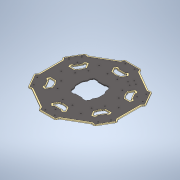
# Autodesk Inventor part: FRAME ATAS
Saved by Autodesk Inventor 2020.2 (Build 242310000, 310)
## iProperties
Created: 2020-03-27
Part Number: FRAME ATAS
Material: Generic
Document SubType Name: Modeling
Designer: Muhyidin
Density: 1 g/cm^3
Appearance: Carbon Fiber
Author: Muhyidin
Autodesk Inventor part; units mm, degrees
(part 1 of 2)
ref_plane "YZ Plane" through (0, 0, 0) normal (1, 0, 0) x (0, 1, 0)
ref_plane "XZ Plane" through (0, 0, 0) normal (0, 1, 0) x (-1, 0, 0)
ref_plane "XY Plane" through (0, 0, 0) normal (0, 0, 1) x (1, 0, 0)
sketch "Sketch1" plane through (0, 0, 0) normal (0, 1, 0) x (-1, 0, 0)
  circle A0 centre (15.3999, -131.0001) radius 1.6
  circle A1 centre (-15.4001, -131) radius 1.6
  line L0 (-50.3385, -87.1889) -> (-60.4808, -89.9065)
  circle A2 centre (-60.4808, -89.9065) radius 1.5
  line L1 (-50.3385, -87.1889) -> (-40.1963, -84.4713)
  line L2 (-50.3385, -87.1889) -> (-47.6209, -97.3311)
  line L3 (-50.3385, -87.1889) -> (-53.0561, -77.0467)
  circle A3 centre (-53.0561, -77.0467) radius 1.5
  circle A4 centre (-40.1963, -84.4713) radius 1.5
  circle A5 centre (-47.6209, -97.3311) radius 1.5
  line L4 (68.5102, -57.3368) -> (53.5102, -83.3176)
  line L5 (83.9102, -30.6632) -> (98.9102, -4.6824)
  line L6 (-68.5102, 57.3368) -> (-53.5102, 83.3176)
  line L7 (-83.9102, 30.6632) -> (-98.9102, 4.6824)
  line L8 (-83.9102, 30.6632) -> (-53.9102, 30.6632) construction
  circle A6 centre (98.9102, -4.6824) radius 1.6
  circle A7 centre (53.5102, -83.3176) radius 1.6
  circle A8 centre (-98.9102, 4.6824) radius 1.6
  circle A9 centre (-53.5102, 83.3176) radius 1.6
  line L9 (53.5102, -83.3176) -> (68.5102, -83.3176) construction
  circle A10 centre (0, 113) radius 1.6
  line L10 (76.2102, -44) -> (97.8609, -56.5)
  line L11 (76.2102, -44) -> (101.2102, -44) construction
  circle A11 centre (97.8609, -56.5) radius 1.6
  line L12 (-76.2102, -44) -> (-97.8609, -56.5)
  line L13 (-76.2102, -44) -> (-51.2102, -44) construction
  circle A12 centre (-97.8609, -56.5) radius 1.6
  line L14 (25, -145) -> (60, -145) construction
  line L15 (0, -138) -> (25, -138)
  line L16 (0, -138) -> (25, -138) construction
  line L17 (0, -138) -> (-25, -138)
  line L18 (0, -138) -> (25, -138) construction
  line L19 (15.4, -138) -> (22.4, -138) construction
  line L20 (-15.4, -138.0001) -> (-8.4, -138.0001) construction
  line L21 (-25, -138) -> (4.9988, -138) construction
  line L22 (-92.0115, -90.6506) -> (-87.0115, -90.6506) construction
  line L23 (-25, -138) -> (-5.0008, -138) construction
  line L24 (-25, -138) -> (-28.4202, -128.6031)
  line L25 (-25, -138) -> (-15, -138) construction
  line L26 (25, -138) -> (28.4201, -128.6031)
  line L27 (132.0114, -47.3494) -> (125.5835, -39.689)
  line L28 (107.0114, -90.6507) -> (97.1633, -88.9142)
  line L29 (111.8115, -82.3369) -> (115.3115, -76.2747) construction
  line L30 (107.0114, -90.6507) -> (117.011, -73.3308) construction
  line L31 (119.5114, -69) -> (107.0114, -90.6507)
  line L32 (107.0114, -90.6507) -> (122.0108, -64.6709) construction
  line L33 (119.5114, -69) -> (132.0114, -47.3494)
  line L34 (119.5114, -69) -> (132.0114, -47.3494) construction
  line L35 (119.5114, -69) -> (132.0114, -47.3494) construction
  circle A13 centre (121.1493, -52.1634) radius 1.6
  circle A14 centre (105.7492, -78.8369) radius 1.6
  line L36 (107.0114, 90.6505) -> (97.1634, 88.914)
  line L37 (132.0114, 47.3493) -> (125.5835, 39.6888)
  line L38 (127.2115, 55.6631) -> (123.7115, 61.7253) construction
  line L39 (132.0114, 47.3493) -> (122.0118, 64.6691) construction
  line L40 (119.5114, 68.9999) -> (132.0114, 47.3493)
  line L41 (132.0114, 47.3493) -> (117.012, 73.329) construction
  line L42 (119.5114, 68.9999) -> (107.0114, 90.6505)
  line L43 (119.5114, 68.9999) -> (107.0114, 90.6505) construction
  line L44 (119.5114, 68.9999) -> (107.0114, 90.6505) construction
  circle A15 centre (105.7494, 78.8366) radius 1.6
  circle A16 centre (121.1493, 52.163) radius 1.6
  line L45 (-25.0001, 137.9998) -> (-28.4202, 128.6029)
  line L46 (24.9999, 137.9998) -> (28.4202, 128.6029)
  line L47 (15.4, 137.9999) -> (8.4, 137.9999) construction
  line L48 (24.9999, 137.9998) -> (5.0007, 137.9998) construction
  line L49 (-0.0001, 137.9998) -> (24.9999, 137.9998)
  line L50 (24.9999, 137.9998) -> (-4.9989, 137.9998) construction
  line L51 (-0.0001, 137.9998) -> (-25.0001, 137.9998)
  line L52 (-0.0001, 137.9998) -> (-25.0001, 137.9998) construction
  line L53 (-0.0001, 137.9998) -> (-25.0001, 137.9998) construction
  circle A17 centre (-15.3999, 130.9999) radius 1.6
  circle A18 centre (15.4, 130.9999) radius 1.6
  line L54 (-132.0115, 47.3492) -> (-125.5836, 39.6889)
  line L55 (-107.0115, 90.6505) -> (-97.1634, 88.914)
  line L56 (-111.8115, 82.3367) -> (-115.3115, 76.2745) construction
  line L57 (-107.0115, 90.6505) -> (-117.0111, 73.3307) construction
  line L58 (-119.5115, 68.9999) -> (-107.0115, 90.6505)
  line L59 (-107.0115, 90.6505) -> (-122.0109, 64.6707) construction
  line L60 (-119.5115, 68.9999) -> (-132.0115, 47.3492)
  line L61 (-119.5115, 68.9999) -> (-132.0115, 47.3492) construction
  line L62 (-119.5115, 68.9999) -> (-132.0115, 47.3492) construction
  circle A19 centre (-121.1493, 52.1632) radius 1.6
  circle A20 centre (-105.7493, 78.8367) radius 1.6
  line L63 (-107.0114, -90.6507) -> (-97.1634, -88.9142)
  line L64 (-132.0114, -47.3494) -> (-125.5836, -39.689)
  line L65 (-127.2115, -55.6633) -> (-123.7115, -61.7255) construction
  line L66 (-132.0114, -47.3494) -> (-122.0118, -64.6693) construction
  line L67 (-119.5114, -69.0001) -> (-132.0114, -47.3494)
  line L68 (-132.0114, -47.3494) -> (-117.012, -73.3292) construction
  line L69 (-119.5114, -69.0001) -> (-107.0114, -90.6507)
  line L70 (-119.5114, -69.0001) -> (-107.0114, -90.6507) construction
  line L71 (-119.5114, -69.0001) -> (-107.0114, -90.6507) construction
  circle A21 centre (-105.7494, -78.8368) radius 1.6
  circle A22 centre (-121.1493, -52.1632) radius 1.6
  line L72 (-28.4202, -128.6031) -> (-97.1634, -88.9142)
  line L73 (97.1633, -88.9142) -> (28.4201, -128.6031)
  line L74 (125.5835, 39.6888) -> (125.5835, -39.689)
  line L75 (28.4202, 128.6029) -> (97.1634, 88.914)
  line L76 (-97.1634, 88.914) -> (-28.4202, 128.6029)
  line L77 (-125.5836, -39.689) -> (-125.5836, 39.6889)
  line L78 (-15.4, -131) -> (42.1, -131) construction
  line L79 (36.5897, -0.0001) -> (36.5897, -10.9001)
  line L80 (36.5897, -0.0001) -> (47.4897, -0.0001) construction
  line L81 (36.5897, -10.9001) -> (30.2097, -21.9505)
  line L82 (36.5897, -10.9001) -> (49.3497, -10.9001) construction
  line L83 (30.2097, -21.9505) -> (30.2097, -30.6505)
  line L84 (30.2097, -21.9505) -> (38.9097, -21.9505) construction
  line L85 (30.2097, -30.6505) -> (23.4386, -38.72)
  line L86 (30.2097, -30.6505) -> (40.7437, -30.6505) construction
  line L87 (23.4386, -38.72) -> (12.9386, -38.72)
  line L88 (12.9386, -38.72) -> (11.0102, -36.4219)
  line L89 (0, -83.2026) -> (6, -83.2026)
  line L90 (6, -83.2026) -> (8.5, -83.2026) construction
  line L91 (6, -83.2026) -> (7.9151, -84.8096)
  line L92 (6, -83.2026) -> (8.5, -83.2026) construction
  line L93 (7.9151, -84.8096) -> (14.9151, -84.8096)
  line L94 (14.9151, -84.8096) -> (24.9151, -102.1301)
  line L95 (14.9151, -90.5569) -> (34.9151, -90.5569) construction
  line L96 (24.9151, -102.1301) -> (19.1301, -109.0245)
  line L97 (24.9151, -115.3493) -> (33.9151, -115.3493) construction
  line L98 (19.1301, -109.0245) -> (13.35, -109.0245)
  line L99 (19.1301, -114.7719) -> (24.9101, -114.7719) construction
  line L100 (13.35, -109.0245) -> (11.1, -105.1274)
  line L101 (13.35, -109.0245) -> (17.85, -109.0245) construction
  line L102 (11.1, -105.1274) -> (0, -105.1274)
  line L103 (0, -83.2026) -> (-6, -83.2026)
  line L104 (-6, -83.2026) -> (-8.5, -83.2026) construction
  line L105 (-6, -83.2026) -> (-7.9151, -84.8096)
  line L106 (-6, -83.2026) -> (-8.5, -83.2026) construction
  line L107 (-7.9151, -84.8096) -> (-14.9151, -84.8096)
  line L108 (-14.9151, -84.8096) -> (-24.9151, -102.1301)
  line L109 (-14.9151, -90.557) -> (-34.9151, -90.557) construction
  line L110 (-24.9151, -102.1301) -> (-19.13, -109.0245)
  line L111 (-19.13, -109.0245) -> (-13.35, -109.0245)
  line L112 (-19.13, -114.7719) -> (-24.91, -114.7719) construction
  line L113 (-13.35, -109.0245) -> (-11.1, -105.1274)
  line L114 (-13.35, -109.0245) -> (-17.85, -109.0245) construction
  line L115 (-11.1, -105.1274) -> (0, -105.1274)
  line L116 (0, -88.9499) -> (0, -36.4219)
  line L117 (0, -86.2026) -> (5.9999, -86.2026)
  line L118 (5.9999, -86.2026) -> (7.532, -87.4882)
  line L119 (5.9999, -86.2026) -> (7.9999, -86.2026) construction
  line L120 (7.532, -87.4882) -> (12.532, -87.4882)
  line L121 (12.532, -87.4882) -> (20.032, -100.4785)
  line L122 (20.032, -100.4785) -> (16.8181, -104.3088)
  line L123 (16.8181, -104.3088) -> (13.8181, -104.3088)
  line L124 (13.8181, -104.3088) -> (12.5681, -102.1437)
  line L125 (12.5681, -102.1437) -> (0, -102.1437)
  line L126 (0, -86.2026) -> (-6, -86.2026)
  line L127 (-6, -86.2026) -> (-7.5321, -87.4882)
  line L128 (-6, -86.2026) -> (-8, -86.2026) construction
  line L129 (-7.5321, -87.4882) -> (-12.5321, -87.4882)
  line L130 (-12.5321, -87.4882) -> (-20.0321, -100.4785)
  line L131 (-20.0321, -100.4785) -> (-16.8181, -104.3088)
  line L132 (-16.8181, -104.3088) -> (-13.8181, -104.3088)
  line L133 (-13.8181, -104.3088) -> (-12.5681, -102.1437)
  line L134 (-12.5681, -102.1437) -> (0, -102.1437)
  line L135 (0, -138) -> (0, -141)
  line L136 (0, -138) -> (3, -138) construction
  line L137 (-25, -138) -> (-22, -138) construction
  line L138 (-25, -138) -> (-20, -138) construction
  line L139 (0, -141) -> (-27.5173, -141)
  line L140 (0, -141) -> (27.5173, -141) construction
  line L141 (-27.5173, -141) -> (-13.8071, -141) construction
  line L142 (-28.4202, -128.6031) -> (-34.2721, -128.6031)
  line L143 (-28.4202, -128.6031) -> (-22.5683, -128.6031) construction
  line L144 (-107.0114, -90.6507) -> (-104.0114, -90.6507) construction
  line L145 (-27.5173, -141) -> (-30.9375, -131.6031)
  line L146 (-27.5173, -141) -> (-17.5173, -141) construction
  line L147 (0, -141) -> (27.5173, -141)
  line L148 (27.5173, -141) -> (13.8071, -141) construction
  line L149 (27.5173, -141) -> (30.9375, -131.6031)
  line L150 (108.3508, -94.3307) -> (98.5028, -92.5942)
  line L151 (122.1095, -70.5) -> (108.3508, -94.3307)
  line L152 (122.1095, -70.5) -> (135.8681, -46.6693) construction
  line L153 (122.1095, -70.5) -> (135.8681, -46.6693)
  line L154 (135.8681, -46.6693) -> (129.4403, -39.0089)
  line L155 (135.8681, 46.6692) -> (129.4402, 39.0088)
  line L156 (122.1095, 70.4999) -> (135.8681, 46.6692)
  line L157 (122.1095, 70.4999) -> (108.3508, 94.3306) construction
  line L158 (122.1095, 70.4999) -> (108.3508, 94.3306)
  line L159 (108.3508, 94.3306) -> (98.5027, 92.5941)
  line L160 (27.5172, 140.9998) -> (30.9374, 131.6029)
  line L161 (-0.0001, 140.9998) -> (27.5172, 140.9998)
  line L162 (-0.0001, 140.9998) -> (-27.5173, 140.9998) construction
  line L163 (-0.0001, 140.9998) -> (-27.5173, 140.9998)
  line L164 (-27.5173, 140.9998) -> (-30.9376, 131.6029)
  line L165 (-108.3509, 94.3305) -> (-98.5028, 92.5941)
  line L166 (-122.1095, 70.4999) -> (-108.3509, 94.3305)
  line L167 (-122.1095, 70.4999) -> (-135.8682, 46.6692) construction
  line L168 (-122.1095, 70.4999) -> (-135.8682, 46.6692)
  line L169 (-135.8682, 46.6692) -> (-129.4403, 39.0087)
  line L170 (-135.8682, -46.6694) -> (-129.4403, -39.0089)
  line L171 (-122.1095, -70.5001) -> (-135.8682, -46.6694)
  line L172 (-122.1095, -70.5001) -> (-108.3509, -94.3307) construction
  line L173 (-122.1095, -70.5001) -> (-108.3509, -94.3307)
  line L174 (-108.3509, -94.3307) -> (-98.5028, -92.5943)
  line L175 (-30.9375, -131.6031) -> (-98.5028, -92.5943)
  line L176 (98.5028, -92.5942) -> (30.9375, -131.6031)
  line L177 (129.4402, 39.0088) -> (129.4403, -39.0089)
  line L178 (30.9374, 131.6029) -> (98.5027, 92.5941)
  line L179 (-98.5028, 92.5941) -> (-30.9376, 131.6029)
  line L180 (-129.4403, -39.0089) -> (-129.4403, 39.0087)
  line L181 (11.0102, -36.4219) -> (0, -36.4219)
  line L182 (-36.5897, -0.0001) -> (-36.5897, -10.9001)
  line L183 (-36.5897, -10.9001) -> (-30.2097, -21.9505)
  line L184 (-36.5897, -10.9001) -> (-49.3497, -10.9001) construction
  line L185 (-30.2097, -21.9505) -> (-30.2097, -30.6505)
  line L186 (-30.2097, -21.9505) -> (-38.9097, -21.9505) construction
  line L187 (-30.2097, -30.6505) -> (-23.4386, -38.72)
  line L188 (-23.4386, -38.72) -> (-12.9386, -38.72)
  line L189 (-12.9386, -38.72) -> (-11.0102, -36.4219)
  line L190 (-11.0102, -36.4219) -> (0, -36.4219)
  line L191 (36.5897, -0.0001) -> (36.5897, 10.8999)
  line L192 (36.5897, 10.8999) -> (30.2097, 21.9504)
  line L193 (36.5897, 10.8999) -> (49.3497, 10.8999) construction
  line L194 (30.2097, 21.9504) -> (30.2097, 30.6504)
  line L195 (30.2097, 21.9504) -> (38.9097, 21.9504) construction
  line L196 (30.2097, 30.6504) -> (23.4386, 38.7199)
  line L197 (23.4386, 38.7199) -> (12.9386, 38.7199)
  line L198 (12.9386, 38.7199) -> (11.0102, 36.4218)
  line L199 (11.0102, 36.4218) -> (0, 36.4218)
  line L200 (-23.4386, 38.7199) -> (-12.9386, 38.7199)
  line L201 (-30.2097, 30.6504) -> (-23.4386, 38.7199)
  line L202 (-11.0102, 36.4218) -> (0, 36.4218)
  line L203 (-12.9386, 38.7199) -> (-11.0102, 36.4218)
  line L204 (-30.2097, 21.9504) -> (-30.2097, 30.6504)
  line L205 (-30.2097, 21.9504) -> (-38.9097, 21.9504) construction
  line L206 (-36.5897, 10.8999) -> (-30.2097, 21.9504)
  line L207 (-36.5897, 10.8999) -> (-49.3497, 10.8999) construction
  line L208 (-36.5897, -0.0001) -> (-36.5897, 10.8999)
  line L209 (-15.4, -131) -> (-15.4, -73.5)
  line L210 (-15.4, -131) -> (42.1, -131) construction
  line L211 (15.3999, -131.0001) -> (15.3999, -73.5001)
  line L212 (15.3999, -73.5001) -> (15.9999, -73.5001)
  line L213 (15.3999, -73.5001) -> (15.9999, -73.5001) construction
  circle A23 centre (15.9999, -73.5001) radius 1.65
  line L214 (-15.4, -73.5) -> (-16.036, -73.5)
  circle A24 centre (-16.0361, -73.5) radius 1.65
  circle A25 centre (55.6348, -50.6377) radius 1.65
  circle A26 centre (71.6528, -22.8937) radius 1.65
  circle A27 centre (71.6708, 22.8623) radius 1.65
  circle A28 centre (55.6529, 50.6063) radius 1.65
  circle A29 centre (16.036, 73.4999) radius 1.65
  circle A30 centre (-15.9999, 73.4999) radius 1.65
  circle A31 centre (-55.6348, 50.6375) radius 1.65
  circle A32 centre (-71.6529, 22.8936) radius 1.65
  circle A33 centre (-71.6709, -22.8624) radius 1.65
  circle A34 centre (-55.6529, -50.6064) radius 1.65
  line L215 (85.4929, -62.1766) -> (91.0429, -52.5637)
  line L216 (82.1749, -61.9562) -> (88.4589, -51.0719)
  line L217 (94.743, -40.1876) -> (88.4589, -51.0719)
  line L218 (96.5929, -42.9508) -> (91.0429, -52.5637)
  line L219 (101.0929, -42.9508) -> (96.5929, -42.9508)
  line L220 (97.243, -40.1876) -> (94.743, -40.1876)
  line L221 (100.9047, -29.488) -> (103.9829, -37.9452)
  line L222 (101.0929, -42.9508) -> (103.3429, -39.0537) construction
  line L223 (103.9829, -37.9452) -> (101.0929, -42.9508)
  line L224 (98.743, -37.5895) -> (97.243, -40.1876)
  line L225 (97.0329, -32.8911) -> (98.743, -37.5895)
  line L226 (80.9047, -29.488) -> (100.9047, -29.488)
  line L227 (82.0329, -32.8911) -> (97.0329, -32.8911)
  line L228 (79.5329, -37.2212) -> (82.0329, -32.8911)
  line L229 (77.4047, -35.5501) -> (80.9047, -29.488)
  line L230 (77.6535, -37.9052) -> (79.5329, -37.2212)
  line L231 (75.0555, -36.4052) -> (77.4047, -35.5501)
  line L232 (75.0555, -36.4052) -> (76.3055, -34.2401) construction
  line L233 (75.0555, -36.4052) -> (76.3055, -34.2401) construction
  line L234 (72.0555, -41.6013) -> (75.0555, -36.4052)
  line L235 (77.6535, -37.9052) -> (78.6535, -36.1732) construction
  line L236 (74.6535, -43.1013) -> (77.6535, -37.9052)
  line L237 (69.0555, -46.7975) -> (67.8055, -48.9625) construction
  line L238 (69.0555, -46.7975) -> (67.8055, -48.9625) construction
  line L239 (72.0555, -41.6013) -> (69.0555, -46.7975)
  line L240 (74.6535, -43.1013) -> (71.6536, -48.2974)
  line L241 (69.0555, -46.7975) -> (69.4896, -49.2595)
  line L242 (71.6536, -48.2974) -> (70.6536, -50.0295) construction
  line L243 (71.6536, -48.2974) -> (72.0008, -50.2671)
  line L244 (69.4896, -49.2595) -> (65.9896, -55.3217)
  line L245 (72.0008, -50.2671) -> (69.5008, -54.5972)
  line L246 (69.5008, -54.5972) -> (77.0008, -67.5876)
  line L247 (65.9896, -55.3217) -> (75.9896, -72.6422)
  line L248 (70.967, -58.1954) -> (60.967, -75.5159) construction
  line L249 (81.9249, -66.7193) -> (83.4249, -64.1213)
  line L250 (84.8529, -71.0793) -> (87.7429, -66.0737)
  line L251 (87.7429, -66.0737) -> (85.4929, -69.9708) construction
  line L252 (87.7429, -66.0737) -> (85.4929, -62.1766)
  line L253 (83.4249, -64.1213) -> (82.1749, -61.9562)
  line L254 (77.0008, -67.5876) -> (81.9249, -66.7193)
  line L255 (75.9896, -72.6422) -> (84.8529, -71.0793)
  line L256 (96.5929, 42.9507) -> (91.0429, 52.5636)
  line L257 (94.743, 40.1874) -> (88.4589, 51.0717)
  line L258 (82.1749, 61.956) -> (88.4589, 51.0717)
  line L259 (85.4929, 62.1765) -> (91.0429, 52.5636)
  line L260 (87.7429, 66.0736) -> (85.4929, 62.1765)
  line L261 (83.4249, 64.1211) -> (82.1749, 61.956)
  line L262 (75.9896, 72.642) -> (84.8529, 71.0793)
  line L263 (87.7429, 66.0736) -> (85.4929, 69.9707) construction
  line L264 (84.8529, 71.0793) -> (87.7429, 66.0736)
  line L265 (81.9249, 66.7192) -> (83.4249, 64.1211)
  line L266 (77.0008, 67.5874) -> (81.9249, 66.7192)
  line L267 (65.9896, 55.3215) -> (75.9896, 72.642)
  line L268 (69.5008, 54.597) -> (77.0008, 67.5874)
  line L269 (72.0008, 50.2669) -> (69.5008, 54.597)
  line L270 (69.4896, 49.2593) -> (65.9896, 55.3215)
  line L271 (71.6536, 48.2973) -> (72.0008, 50.2669)
  line L272 (69.0555, 46.7973) -> (69.4896, 49.2593)
  line L273 (69.0555, 46.7973) -> (67.8054, 48.9624) construction
  line L274 (69.0555, 46.7973) -> (67.8055, 48.9624) construction
  line L275 (72.0555, 41.6012) -> (69.0555, 46.7973)
  line L276 (71.6536, 48.2973) -> (70.6536, 50.0293) construction
  line L277 (74.6535, 43.1012) -> (71.6536, 48.2973)
  line L278 (75.0555, 36.4051) -> (76.3055, 34.24) construction
  line L279 (75.0555, 36.4051) -> (76.3055, 34.24) construction
  line L280 (72.0555, 41.6012) -> (75.0555, 36.4051)
  line L281 (74.6535, 43.1012) -> (77.6535, 37.9051)
  line L282 (75.0555, 36.4051) -> (77.4047, 35.55)
  line L283 (77.6535, 37.9051) -> (78.6535, 36.173) construction
  line L284 (77.6535, 37.9051) -> (79.5329, 37.221)
  line L285 (77.4047, 35.55) -> (80.9047, 29.4879)
  line L286 (79.5329, 37.221) -> (82.0329, 32.8909)
  line L287 (82.0329, 32.8909) -> (97.0329, 32.8909)
  line L288 (80.9047, 29.4879) -> (100.9047, 29.4879)
  line L289 (85.8821, 32.3615) -> (95.8821, 15.041) construction
  line L290 (98.743, 37.5894) -> (97.243, 40.1874)
  line L291 (103.9829, 37.9451) -> (101.0929, 42.9507)
  line L292 (101.0929, 42.9507) -> (103.3429, 39.0536) construction
  line L293 (101.0929, 42.9507) -> (96.5929, 42.9507)
  line L294 (97.243, 40.1874) -> (94.743, 40.1874)
  line L295 (97.0329, 32.8909) -> (98.743, 37.5894)
  line L296 (100.9047, 29.4879) -> (103.9829, 37.9451)
  line L297 (11.0999, 105.1272) -> (-0.0001, 105.1272)
  line L298 (12.5681, 102.1435) -> (0, 102.1435)
  line L299 (-12.5681, 102.1435) -> (0, 102.1435)
  line L300 (-11.1001, 105.1272) -> (-0.0001, 105.1272)
  line L301 (-13.3501, 109.0244) -> (-11.1001, 105.1272)
  line L302 (-13.8181, 104.3086) -> (-12.5681, 102.1435)
  line L303 (-24.9151, 102.1299) -> (-19.1301, 109.0244)
  line L304 (-13.3501, 109.0244) -> (-17.8501, 109.0244) construction
  line L305 (-19.1301, 109.0244) -> (-13.3501, 109.0244)
  line L306 (-16.8181, 104.3086) -> (-13.8181, 104.3086)
  line L307 (-20.0321, 100.4784) -> (-16.8181, 104.3086)
  line L308 (-14.9151, 84.8094) -> (-24.9151, 102.1299)
  line L309 (-12.5321, 87.488) -> (-20.0321, 100.4784)
  line L310 (-7.5321, 87.488) -> (-12.5321, 87.488)
  line L311 (-7.9151, 84.8094) -> (-14.9151, 84.8094)
  line L312 (-6, 86.2024) -> (-7.5321, 87.488)
  line L313 (-6, 83.2024) -> (-7.9151, 84.8094)
  line L314 (-6, 83.2024) -> (-8.5001, 83.2024) construction
  line L315 (-6, 83.2024) -> (-8.5, 83.2024) construction
  line L316 (0, 83.2024) -> (-6, 83.2024)
  line L317 (-6, 86.2024) -> (-8, 86.2024) construction
  line L318 (0, 86.2024) -> (-6, 86.2024)
  line L319 (5.9999, 83.2025) -> (8.4999, 83.2025) construction
  line L320 (5.9999, 83.2025) -> (8.4999, 83.2025) construction
  line L321 (0, 83.2024) -> (5.9999, 83.2025)
  line L322 (0, 86.2024) -> (5.9999, 86.2024)
  line L323 (5.9999, 83.2025) -> (7.915, 84.8094)
  line L324 (5.9999, 86.2024) -> (7.9999, 86.2024) construction
  line L325 (5.9999, 86.2024) -> (7.532, 87.488)
  line L326 (7.915, 84.8094) -> (14.915, 84.8094)
  line L327 (7.532, 87.488) -> (12.532, 87.488)
  line L328 (12.532, 87.488) -> (20.032, 100.4784)
  line L329 (14.915, 84.8094) -> (24.915, 102.13)
  line L330 (14.915, 90.5568) -> (34.915, 90.5568) construction
  line L331 (16.8181, 104.3086) -> (13.8181, 104.3086)
  line L332 (19.13, 109.0244) -> (13.3499, 109.0244)
  line L333 (13.3499, 109.0244) -> (17.8499, 109.0244) construction
  line L334 (13.3499, 109.0244) -> (11.0999, 105.1272)
  line L335 (13.8181, 104.3086) -> (12.5681, 102.1435)
  line L336 (20.032, 100.4784) -> (16.8181, 104.3086)
  line L337 (24.915, 102.13) -> (19.13, 109.0244)
  line L338 (-85.493, 62.1764) -> (-91.043, 52.5635)
  line L339 (-82.1749, 61.956) -> (-88.459, 51.0717)
  line L340 (-94.743, 40.1874) -> (-88.459, 51.0717)
  line L341 (-96.593, 42.9507) -> (-91.043, 52.5635)
  line L342 (-101.093, 42.9507) -> (-96.593, 42.9507)
  line L343 (-97.243, 40.1874) -> (-94.743, 40.1874)
  line L344 (-100.9047, 29.4878) -> (-103.983, 37.945)
  line L345 (-101.093, 42.9507) -> (-103.343, 39.0535) construction
  line L346 (-103.983, 37.945) -> (-101.093, 42.9507)
  line L347 (-98.743, 37.5894) -> (-97.243, 40.1874)
  line L348 (-97.0329, 32.8909) -> (-98.743, 37.5894)
  line L349 (-80.9047, 29.4878) -> (-100.9047, 29.4878)
  line L350 (-82.0329, 32.8909) -> (-97.0329, 32.8909)
  line L351 (-79.5329, 37.221) -> (-82.0329, 32.8909)
  line L352 (-77.4047, 35.55) -> (-80.9047, 29.4878)
  line L353 (-77.6536, 37.9051) -> (-79.5329, 37.221)
  line L354 (-75.0555, 36.405) -> (-77.4047, 35.55)
  line L355 (-75.0555, 36.405) -> (-76.3055, 34.2399) construction
  line L356 (-75.0555, 36.405) -> (-76.3055, 34.24) construction
  line L357 (-72.0555, 41.6012) -> (-75.0555, 36.405)
  line L358 (-77.6536, 37.9051) -> (-78.6536, 36.173) construction
  line L359 (-74.6536, 43.1012) -> (-77.6536, 37.9051)
  line L360 (-69.0556, 46.7973) -> (-67.8056, 48.9624) construction
  line L361 (-69.0556, 46.7973) -> (-67.8056, 48.9624) construction
  line L362 (-72.0555, 41.6012) -> (-69.0556, 46.7973)
  line L363 (-74.6536, 43.1012) -> (-71.6536, 48.2973)
  line L364 (-69.0556, 46.7973) -> (-69.4897, 49.2593)
  line L365 (-71.6536, 48.2973) -> (-70.6536, 50.0293) construction
  line L366 (-71.6536, 48.2973) -> (-72.0009, 50.2669)
  line L367 (-69.4897, 49.2593) -> (-65.9897, 55.3215)
  line L368 (-72.0009, 50.2669) -> (-69.5009, 54.597)
  line L369 (-69.5009, 54.597) -> (-77.0009, 67.5874)
  line L370 (-65.9897, 55.3215) -> (-75.9897, 72.642)
  line L371 (-70.9671, 58.1952) -> (-60.9671, 75.5157) construction
  line L372 (-81.9249, 66.7192) -> (-83.4249, 64.1211)
  line L373 (-84.853, 71.0792) -> (-87.743, 66.0735)
  line L374 (-87.743, 66.0735) -> (-85.493, 69.9707) construction
  line L375 (-87.743, 66.0735) -> (-85.493, 62.1764)
  line L376 (-83.4249, 64.1211) -> (-82.1749, 61.956)
  line L377 (-77.0009, 67.5874) -> (-81.9249, 66.7192)
  line L378 (-75.9897, 72.642) -> (-84.853, 71.0792)
  line L379 (-96.5929, -42.9509) -> (-91.0429, -52.5638)
  line L380 (-94.743, -40.1876) -> (-88.459, -51.0719)
  line L381 (-82.1749, -61.9562) -> (-88.459, -51.0719)
  line L382 (-85.4929, -62.1767) -> (-91.0429, -52.5638)
  line L383 (-87.7429, -66.0738) -> (-85.4929, -62.1767)
  line L384 (-83.4249, -64.1213) -> (-82.1749, -61.9562)
  line L385 (-75.9896, -72.6422) -> (-84.8529, -71.0794)
  line L386 (-87.7429, -66.0738) -> (-85.4929, -69.9709) construction
  line L387 (-84.8529, -71.0794) -> (-87.7429, -66.0738)
  line L388 (-81.9249, -66.7193) -> (-83.4249, -64.1213)
  line L389 (-77.0009, -67.5876) -> (-81.9249, -66.7193)
  line L390 (-65.9896, -55.3217) -> (-75.9896, -72.6422)
  line L391 (-69.5009, -54.5972) -> (-77.0009, -67.5876)
  line L392 (-72.0009, -50.2671) -> (-69.5009, -54.5972)
  line L393 (-69.4896, -49.2595) -> (-65.9896, -55.3217)
  line L394 (-71.6536, -48.2974) -> (-72.0009, -50.2671)
  line L395 (-69.0555, -46.7975) -> (-69.4896, -49.2595)
  line L396 (-69.0555, -46.7975) -> (-67.8055, -48.9626) construction
  line L397 (-69.0555, -46.7975) -> (-67.8055, -48.9625) construction
  line L398 (-72.0555, -41.6013) -> (-69.0555, -46.7975)
  line L399 (-71.6536, -48.2974) -> (-70.6536, -50.0295) construction
  line L400 (-74.6536, -43.1013) -> (-71.6536, -48.2974)
  line L401 (-75.0555, -36.4052) -> (-76.3055, -34.2402) construction
  line L402 (-75.0555, -36.4052) -> (-76.3055, -34.2402) construction
  line L403 (-72.0555, -41.6013) -> (-75.0555, -36.4052)
  line L404 (-74.6536, -43.1013) -> (-77.6536, -37.9052)
  line L405 (-75.0555, -36.4052) -> (-77.4048, -35.5502)
  line L406 (-77.6536, -37.9052) -> (-78.6536, -36.1732) construction
  line L407 (-77.6536, -37.9052) -> (-79.5329, -37.2212)
  line L408 (-77.4048, -35.5502) -> (-80.9048, -29.488)
  line L409 (-79.5329, -37.2212) -> (-82.0329, -32.8911)
  line L410 (-82.0329, -32.8911) -> (-97.0329, -32.8911)
  line L411 (-80.9048, -29.488) -> (-100.9048, -29.488)
  line L412 (-85.8821, -32.3617) -> (-95.8821, -15.0412) construction
  line L413 (-98.743, -37.5895) -> (-97.243, -40.1876)
  line L414 (-103.9829, -37.9453) -> (-101.0929, -42.9509)
  line L415 (-101.0929, -42.9509) -> (-103.3429, -39.0538) construction
  line L416 (-101.0929, -42.9509) -> (-96.5929, -42.9509)
  line L417 (-97.243, -40.1876) -> (-94.743, -40.1876)
  line L418 (-97.0329, -32.8911) -> (-98.743, -37.5895)
  line L419 (-100.9048, -29.488) -> (-103.9829, -37.9453)
  point P0 (0, -0.0001)
  point P1 (-50.3385, -87.1889)
  point P2 (-50.3385, -87.1889)
  point P3 (-50.3385, -87.1889)
  point P4 (-50.3385, -87.1889)
  point P5 (-50.3385, -87.1889)
  point P6 (28.4201, -128.6031)
  point P7 (-28.4202, 128.6029)
  dimension "d427" = 3.2
  dimension "d428" = 3.2
  dimension "d473" = 10.5
  dimension "d474" = 3
  dimension "d479" = 10.5
  dimension "d480" = 10.5
  dimension "d481" = 10.5
  dimension "d486" = 3
  dimension "d491" = 3
  dimension "d496" = 3
  dimension "d497" = 30
  dimension "d498" = 30
  dimension "d499" = 30
  dimension "d500" = 30
  dimension "d501" = 120
  dimension "d597" = 25
  dimension "d598" = 30
  dimension "d603" = 25
  dimension "d604" = 150
  dimension "d625" = 0
  dimension "d627" = 180
  dimension "d646" = 10
  dimension "d647" = 110
  dimension "d650" = 360
  dimension "d655" = 360
  dimension "d672" = 10.9
  dimension "d673" = 90
  dimension "d674" = 12.76
  dimension "d675" = 120
  dimension "d676" = 8.7
  dimension "d677" = 90
  dimension "d678" = 10.534
  dimension "d679" = 130
  dimension "d680" = 10.5
  dimension "d681" = 3
  dimension "d684" = 6
  dimension "d687" = 2.5
  dimension "d688" = 40
  dimension "d689" = 7
  dimension "d690" = 20
  dimension "d691" = 60
  dimension "d692" = 9
  dimension "d693" = 129.999
  dimension "d695" = 180
  dimension "d696" = 4.5
  dimension "d697" = 120
  dimension "d705" = 3
  dimension "d706" = 2
  dimension "d707" = 40
  dimension "d708" = 5
  dimension "d709" = 140
  dimension "d710" = 15
  dimension "d711" = 120
  dimension "d712" = 5
  dimension "d713" = 110
  dimension "d714" = 3
  dimension "d715" = 130
  dimension "d716" = 2.5
  dimension "d717" = 120
  dimension "d722" = 3
  dimension "d723" = 90
  dimension "d729" = 180
  dimension "d731" = 180
  dimension "d735" = 10
  constraints: 840 end point, 45 horizontal, 35 centre point, 22 equal length, 4 vertical, 3 parallel, 3 perpendicular, 2 coincident, 2 symmetric about line, 768 other
  measures "d427" diameter of A0
  measures "d428" diameter of A1
  measures "d473" distance of L0.end L0.start
  measures "d474" diameter of A2
  measures "d479" distance of L1.start L1.end
  measures "d480" distance of L1.start L2.end
  measures "d481" distance of L1.start L3.end
  measures "d486" diameter of A3
  measures "d491" diameter of A4
  measures "d496" diameter of A5
  measures "d497" distance of L4.start L4.end
  measures "d498" distance of L5.start L5.end
  measures "d499" distance of L6.start L6.end
  measures "d500" distance of L7.start L7.end
  measures "d501" angle of L7 L8
  measures "d597" distance of L10.start L10.end
  measures "d598" angle of L10 L11
  measures "d603" distance of L12.start L12.end
  measures "d604" angle of L12 L13
  measures "d625" distance between parallel lines of L15 L16
  measures "d627" angle of L17 L18
  measures "d646" distance of L17.end L24.end
  measures "d647" angle of L25 L24
  measures "d672" distance of L79.start L79.end
  measures "d673" angle of L79 L80
  measures "d674" distance of L79.end L81.end
  measures "d675" angle of L81 L82
  measures "d676" distance of L81.end L83.end
  measures "d677" angle of L83 L84
  measures "d678" distance of L83.end L85.end
  measures "d679" angle of L85 L86
  measures "d680" distance of L85.end L87.end
  measures "d681" distance of L87.end L88.end
  measures "d684" distance of L89.start L89.end
  measures "d687" distance of L89.end L91.end
  measures "d688" angle of L91 L92
  measures "d689" distance of L91.end L93.end
  measures "d690" distance of L93.end L94.end
  measures "d691" angle of L94 L95
  measures "d692" distance of L94.end L96.end
  measures "d693" angle of L96 L97
  measures "d695" angle of L98 L99
  measures "d696" distance of L98.end L100.end
  measures "d697" angle of L101 L100
  measures "d705" distance of L89.start L117.start
  measures "d706" distance of L117.end L118.end
  measures "d707" angle of L118 L119
  measures "d708" distance of L118.end L120.end
  measures "d709" angle of L120 L118
  measures "d710" distance of L120.end L121.end
  measures "d711" angle of L120 L121
  measures "d712" distance of L121.end L122.end
  measures "d713" angle of L121 L122
  measures "d714" distance of L122.end L123.end
  measures "d715" angle of L122 L123
  measures "d716" distance of L123.end L124.end
  measures "d717" angle of L123 L124
  measures "d722" distance of L15.start L135.end
  measures "d723" angle of L135 L136
  measures "d729" angle of L139 L140
  measures "d731" angle of L142 L143
  measures "d735" distance of L139.end L145.end
extrude "Extrusion11" add sketch "Sketch1" along normal blind 3 contours L17 L24 L72 L63 L69 L67 L64 L77 L54 L60 L58 L55 L76 L45 L51 L49 L46 L75 L36 L42 L40 L37 L74 L27 L33 L31 L28 L73 L26 L15
sketch "Sketch3" plane through (0, 3, 0) normal (0, 1, 0) x (1, 0, 0)
  circle A0 centre (15.3999, -131.0001) radius 1.6
  circle A1 centre (-15.4001, -131) radius 1.6
  line L0 (-83.9102, 30.6632) -> (-53.9102, 30.6632) construction
  line L1 (76.2102, -44) -> (101.2102, -44) construction
  line L2 (-76.2102, -44) -> (-51.2102, -44) construction
  line L3 (25, -145) -> (60, -145) construction
  line L4 (0, -138) -> (25, -138)
  line L5 (0, -138) -> (25, -138) construction
  line L6 (0, -138) -> (-25, -138)
  line L7 (0, -138) -> (25, -138) construction
  line L8 (15.4, -138) -> (22.4, -138) construction
  line L9 (-15.4, -138.0001) -> (-8.4, -138.0001) construction
  line L10 (-25, -138) -> (4.9988, -138) construction
  line L11 (-92.0115, -90.6506) -> (-87.0115, -90.6506) construction
  line L12 (-25, -138) -> (-5.0008, -138) construction
  line L13 (-25, -138) -> (-28.4202, -128.6031)
  line L14 (-25, -138) -> (-15, -138) construction
  line L15 (25, -138) -> (28.4201, -128.6031)
  line L16 (132.0114, -47.3494) -> (125.5835, -39.689)
  line L17 (107.0114, -90.6507) -> (97.1633, -88.9142)
  line L18 (111.8115, -82.3369) -> (115.3115, -76.2747) construction
  line L19 (107.0114, -90.6507) -> (117.011, -73.3308) construction
  line L20 (119.5114, -69) -> (107.0114, -90.6507)
  line L21 (107.0114, -90.6507) -> (122.0108, -64.6709) construction
  line L22 (119.5114, -69) -> (132.0114, -47.3494)
  line L23 (119.5114, -69) -> (132.0114, -47.3494) construction
  line L24 (119.5114, -69) -> (132.0114, -47.3494) construction
  circle A2 centre (121.1493, -52.1634) radius 1.6
  circle A3 centre (105.7492, -78.8369) radius 1.6
  line L25 (107.0114, 90.6505) -> (97.1634, 88.914)
  line L26 (132.0114, 47.3493) -> (125.5835, 39.6888)
  line L27 (127.2115, 55.6631) -> (123.7115, 61.7253) construction
  line L28 (132.0114, 47.3493) -> (122.0118, 64.6691) construction
  line L29 (119.5114, 68.9999) -> (132.0114, 47.3493)
  line L30 (132.0114, 47.3493) -> (117.012, 73.329) construction
  line L31 (119.5114, 68.9999) -> (107.0114, 90.6505)
  line L32 (119.5114, 68.9999) -> (107.0114, 90.6505) construction
  line L33 (119.5114, 68.9999) -> (107.0114, 90.6505) construction
  circle A4 centre (105.7494, 78.8366) radius 1.6
  circle A5 centre (121.1493, 52.163) radius 1.6
  line L34 (-25.0001, 137.9998) -> (-28.4202, 128.6029)
  line L35 (24.9999, 137.9998) -> (28.4202, 128.6029)
  line L36 (15.4, 137.9999) -> (8.4, 137.9999) construction
  line L37 (24.9999, 137.9998) -> (5.0007, 137.9998) construction
  line L38 (-0.0001, 137.9998) -> (24.9999, 137.9998)
  line L39 (24.9999, 137.9998) -> (-4.9989, 137.9998) construction
  line L40 (-0.0001, 137.9998) -> (-25.0001, 137.9998)
  line L41 (-0.0001, 137.9998) -> (-25.0001, 137.9998) construction
  line L42 (-0.0001, 137.9998) -> (-25.0001, 137.9998) construction
  circle A6 centre (-15.3999, 130.9999) radius 1.6
  circle A7 centre (15.4, 130.9999) radius 1.6
  line L43 (-132.0115, 47.3492) -> (-125.5836, 39.6889)
  line L44 (-107.0115, 90.6505) -> (-97.1634, 88.914)
  line L45 (-111.8115, 82.3367) -> (-115.3115, 76.2745) construction
  line L46 (-107.0115, 90.6505) -> (-117.0111, 73.3307) construction
  line L47 (-119.5115, 68.9999) -> (-107.0115, 90.6505)
  line L48 (-107.0115, 90.6505) -> (-122.0109, 64.6707) construction
  line L49 (-119.5115, 68.9999) -> (-132.0115, 47.3492)
  line L50 (-119.5115, 68.9999) -> (-132.0115, 47.3492) construction
  line L51 (-119.5115, 68.9999) -> (-132.0115, 47.3492) construction
  circle A8 centre (-121.1493, 52.1632) radius 1.6
  circle A9 centre (-105.7493, 78.8367) radius 1.6
  line L52 (-107.0114, -90.6507) -> (-97.1634, -88.9142)
  line L53 (-132.0114, -47.3494) -> (-125.5836, -39.689)
  line L54 (-127.2115, -55.6633) -> (-123.7115, -61.7255) construction
  line L55 (-132.0114, -47.3494) -> (-122.0118, -64.6693) construction
  line L56 (-119.5114, -69.0001) -> (-132.0114, -47.3494)
  line L57 (-132.0114, -47.3494) -> (-117.012, -73.3292) construction
  line L58 (-119.5114, -69.0001) -> (-107.0114, -90.6507)
  line L59 (-119.5114, -69.0001) -> (-107.0114, -90.6507) construction
  line L60 (-119.5114, -69.0001) -> (-107.0114, -90.6507) construction
  circle A10 centre (-105.7494, -78.8368) radius 1.6
  circle A11 centre (-121.1493, -52.1632) radius 1.6
  line L61 (-28.4202, -128.6031) -> (-97.1634, -88.9142)
  line L62 (97.1633, -88.9142) -> (28.4201, -128.6031)
  line L63 (125.5835, 39.6888) -> (125.5835, -39.689)
  line L64 (28.4202, 128.6029) -> (97.1634, 88.914)
  line L65 (-97.1634, 88.914) -> (-28.4202, 128.6029)
  line L66 (-125.5836, -39.689) -> (-125.5836, 39.6889)
  line L67 (-15.4, -131) -> (42.1, -131) construction
  line L68 (36.5897, -0.0001) -> (36.5897, -10.9001)
  line L69 (36.5897, -0.0001) -> (47.4897, -0.0001) construction
  line L70 (36.5897, -10.9001) -> (30.2097, -21.9505)
  line L71 (36.5897, -10.9001) -> (49.3497, -10.9001) construction
  line L72 (30.2097, -21.9505) -> (30.2097, -30.6505)
  line L73 (30.2097, -21.9505) -> (38.9097, -21.9505) construction
  line L74 (30.2097, -30.6505) -> (23.4386, -38.72)
  line L75 (30.2097, -30.6505) -> (40.7437, -30.6505) construction
  line L76 (23.4386, -38.72) -> (12.9386, -38.72)
  line L77 (12.9386, -38.72) -> (11.0102, -36.4219)
  line L78 (0, -83.2026) -> (6, -83.2026)
  line L79 (6, -83.2026) -> (8.5, -83.2026) construction
  line L80 (6, -83.2026) -> (7.9151, -84.8096)
  line L81 (6, -83.2026) -> (8.5, -83.2026) construction
  line L82 (7.9151, -84.8096) -> (14.9151, -84.8096)
  line L83 (14.9151, -84.8096) -> (24.9151, -102.1301)
  line L84 (14.9151, -90.5569) -> (34.9151, -90.5569) construction
  line L85 (24.9151, -102.1301) -> (19.1301, -109.0245)
  line L86 (24.9151, -115.3493) -> (33.9151, -115.3493) construction
  line L87 (19.1301, -109.0245) -> (13.35, -109.0245)
  line L88 (19.1301, -114.7719) -> (24.9101, -114.7719) construction
  line L89 (13.35, -109.0245) -> (11.1, -105.1274)
  line L90 (13.35, -109.0245) -> (17.85, -109.0245) construction
  line L91 (11.1, -105.1274) -> (0, -105.1274)
  line L92 (-11.1, -105.1274) -> (0, -105.1274)
  line L93 (-13.35, -109.0245) -> (-17.85, -109.0245) construction
  line L94 (-19.13, -109.0245) -> (-13.35, -109.0245)
  line L95 (0, -83.2026) -> (-6, -83.2026)
  line L96 (-6, -83.2026) -> (-7.9151, -84.8096)
  line L97 (-6, -83.2026) -> (-8.5, -83.2026) construction
  line L98 (-6, -83.2026) -> (-8.5, -83.2026) construction
  line L99 (-7.9151, -84.8096) -> (-14.9151, -84.8096)
  line L100 (-19.13, -114.7719) -> (-24.91, -114.7719) construction
  line L101 (-24.9151, -102.1301) -> (-19.13, -109.0245)
  line L102 (-14.9151, -84.8096) -> (-24.9151, -102.1301)
  line L103 (-14.9151, -90.557) -> (-34.9151, -90.557) construction
  line L104 (-13.35, -109.0245) -> (-11.1, -105.1274)
  line L105 (0, -88.9499) -> (0, -36.4219)
  line L106 (0, -86.2026) -> (5.9999, -86.2026)
  line L107 (5.9999, -86.2026) -> (7.532, -87.4882)
  line L108 (5.9999, -86.2026) -> (7.9999, -86.2026) construction
  line L109 (7.532, -87.4882) -> (12.532, -87.4882)
  line L110 (12.532, -87.4882) -> (20.032, -100.4785)
  line L111 (20.032, -100.4785) -> (16.8181, -104.3088)
  line L112 (16.8181, -104.3088) -> (13.8181, -104.3088)
  line L113 (13.8181, -104.3088) -> (12.5681, -102.1437)
  line L114 (12.5681, -102.1437) -> (0, -102.1437)
  line L115 (-6, -86.2026) -> (-8, -86.2026) construction
  line L116 (0, -86.2026) -> (-6, -86.2026)
  line L117 (-7.5321, -87.4882) -> (-12.5321, -87.4882)
  line L118 (-6, -86.2026) -> (-7.5321, -87.4882)
  line L119 (-12.5321, -87.4882) -> (-20.0321, -100.4785)
  line L120 (-13.8181, -104.3088) -> (-12.5681, -102.1437)
  line L121 (-16.8181, -104.3088) -> (-13.8181, -104.3088)
  line L122 (-20.0321, -100.4785) -> (-16.8181, -104.3088)
  line L123 (-12.5681, -102.1437) -> (0, -102.1437)
  line L124 (0, -138) -> (0, -141)
  line L125 (0, -138) -> (3, -138) construction
  line L126 (-25, -138) -> (-22, -138) construction
  line L127 (-25, -138) -> (-20, -138) construction
  line L128 (0, -141) -> (-27.5173, -141)
  line L129 (0, -141) -> (27.5173, -141) construction
  line L130 (-27.5173, -141) -> (-13.8071, -141) construction
  line L131 (-28.4202, -128.6031) -> (-34.2721, -128.6031)
  line L132 (-28.4202, -128.6031) -> (-22.5683, -128.6031) construction
  line L133 (-107.0114, -90.6507) -> (-104.0114, -90.6507) construction
  line L134 (-27.5173, -141) -> (-30.9375, -131.6031)
  line L135 (-27.5173, -141) -> (-17.5173, -141) construction
  line L136 (0, -141) -> (27.5173, -141)
  line L137 (27.5173, -141) -> (13.8071, -141) construction
  line L138 (27.5173, -141) -> (30.9375, -131.6031)
  line L139 (108.3508, -94.3307) -> (98.5028, -92.5942)
  line L140 (122.1095, -70.5) -> (108.3508, -94.3307)
  line L141 (122.1095, -70.5) -> (135.8681, -46.6693) construction
  line L142 (122.1095, -70.5) -> (135.8681, -46.6693)
  line L143 (135.8681, -46.6693) -> (129.4403, -39.0089)
  line L144 (135.8681, 46.6692) -> (129.4402, 39.0088)
  line L145 (122.1095, 70.4999) -> (135.8681, 46.6692)
  line L146 (122.1095, 70.4999) -> (108.3508, 94.3306) construction
  line L147 (122.1095, 70.4999) -> (108.3508, 94.3306)
  line L148 (108.3508, 94.3306) -> (98.5027, 92.5941)
  line L149 (27.5172, 140.9998) -> (30.9374, 131.6029)
  line L150 (-0.0001, 140.9998) -> (27.5172, 140.9998)
  line L151 (-0.0001, 140.9998) -> (-27.5173, 140.9998) construction
  line L152 (-0.0001, 140.9998) -> (-27.5173, 140.9998)
  line L153 (-27.5173, 140.9998) -> (-30.9376, 131.6029)
  line L154 (-108.3509, 94.3305) -> (-98.5028, 92.5941)
  line L155 (-122.1095, 70.4999) -> (-108.3509, 94.3305)
  line L156 (-122.1095, 70.4999) -> (-135.8682, 46.6692) construction
  line L157 (-122.1095, 70.4999) -> (-135.8682, 46.6692)
  line L158 (-135.8682, 46.6692) -> (-129.4403, 39.0087)
  line L159 (-135.8682, -46.6694) -> (-129.4403, -39.0089)
  line L160 (-122.1095, -70.5001) -> (-135.8682, -46.6694)
  line L161 (-122.1095, -70.5001) -> (-108.3509, -94.3307) construction
  line L162 (-122.1095, -70.5001) -> (-108.3509, -94.3307)
  line L163 (-108.3509, -94.3307) -> (-98.5028, -92.5943)
  line L164 (-30.9375, -131.6031) -> (-98.5028, -92.5943)
  line L165 (98.5028, -92.5942) -> (30.9375, -131.6031)
  line L166 (129.4402, 39.0088) -> (129.4403, -39.0089)
  line L167 (30.9374, 131.6029) -> (98.5027, 92.5941)
  line L168 (-98.5028, 92.5941) -> (-30.9376, 131.6029)
  line L169 (-129.4403, -39.0089) -> (-129.4403, 39.0087)
  line L170 (11.0102, -36.4219) -> (0, -36.4219)
  line L171 (-12.9386, -38.72) -> (-11.0102, -36.4219)
  line L172 (-11.0102, -36.4219) -> (0, -36.4219)
  line L173 (-23.4386, -38.72) -> (-12.9386, -38.72)
  line L174 (-30.2097, -30.6505) -> (-23.4386, -38.72)
  line L175 (-30.2097, -21.9505) -> (-30.2097, -30.6505)
  line L176 (-30.2097, -21.9505) -> (-38.9097, -21.9505) construction
  line L177 (-36.5897, -10.9001) -> (-30.2097, -21.9505)
  line L178 (-36.5897, -0.0001) -> (-36.5897, -10.9001)
  line L179 (-36.5897, -10.9001) -> (-49.3497, -10.9001) construction
  line L180 (23.4386, 38.7199) -> (12.9386, 38.7199)
  line L181 (30.2097, 30.6504) -> (23.4386, 38.7199)
  line L182 (11.0102, 36.4218) -> (0, 36.4218)
  line L183 (12.9386, 38.7199) -> (11.0102, 36.4218)
  line L184 (30.2097, 21.9504) -> (30.2097, 30.6504)
  line L185 (30.2097, 21.9504) -> (38.9097, 21.9504) construction
  line L186 (36.5897, 10.8999) -> (30.2097, 21.9504)
  line L187 (36.5897, 10.8999) -> (49.3497, 10.8999) construction
  line L188 (36.5897, -0.0001) -> (36.5897, 10.8999)
  line L189 (-36.5897, 10.8999) -> (-49.3497, 10.8999) construction
  line L190 (-36.5897, -0.0001) -> (-36.5897, 10.8999)
  line L191 (-30.2097, 21.9504) -> (-38.9097, 21.9504) construction
  line L192 (-36.5897, 10.8999) -> (-30.2097, 21.9504)
  line L193 (-30.2097, 21.9504) -> (-30.2097, 30.6504)
  line L194 (-30.2097, 30.6504) -> (-23.4386, 38.7199)
  line L195 (-23.4386, 38.7199) -> (-12.9386, 38.7199)
  line L196 (-12.9386, 38.7199) -> (-11.0102, 36.4218)
  line L197 (-11.0102, 36.4218) -> (0, 36.4218)
  line L198 (-15.4, -131) -> (-15.4, -73.5)
  line L199 (-15.4, -131) -> (42.1, -131) construction
  line L200 (15.3999, -131.0001) -> (15.3999, -73.5001)
  line L201 (15.3999, -73.5001) -> (15.9999, -73.5001)
  line L202 (15.3999, -73.5001) -> (15.9999, -73.5001) construction
  circle A12 centre (15.9999, -73.5001) radius 1.65
  line L203 (-15.4, -73.5) -> (-16.036, -73.5)
  circle A13 centre (-16.0361, -73.5) radius 1.65
  line L204 (85.4929, -62.1766) -> (91.0429, -52.5637)
  line L205 (82.1749, -61.9562) -> (88.4589, -51.0719)
  line L206 (94.743, -40.1876) -> (88.4589, -51.0719)
  line L207 (96.5929, -42.9508) -> (91.0429, -52.5637)
  line L208 (101.0929, -42.9508) -> (96.5929, -42.9508)
  line L209 (97.243, -40.1876) -> (94.743, -40.1876)
  line L210 (100.9047, -29.488) -> (103.9829, -37.9452)
  line L211 (101.0929, -42.9508) -> (103.3429, -39.0537) construction
  line L212 (103.9829, -37.9452) -> (101.0929, -42.9508)
  line L213 (98.743, -37.5895) -> (97.243, -40.1876)
  line L214 (97.0329, -32.8911) -> (98.743, -37.5895)
  line L215 (80.9047, -29.488) -> (100.9047, -29.488)
  line L216 (82.0329, -32.8911) -> (97.0329, -32.8911)
  line L217 (79.5329, -37.2212) -> (82.0329, -32.8911)
  line L218 (77.4047, -35.5501) -> (80.9047, -29.488)
  line L219 (77.6535, -37.9052) -> (79.5329, -37.2212)
  line L220 (75.0555, -36.4052) -> (77.4047, -35.5501)
  line L221 (75.0555, -36.4052) -> (76.3055, -34.2401) construction
  line L222 (75.0555, -36.4052) -> (76.3055, -34.2401) construction
  line L223 (72.0555, -41.6013) -> (75.0555, -36.4052)
  line L224 (77.6535, -37.9052) -> (78.6535, -36.1732) construction
  line L225 (74.6535, -43.1013) -> (77.6535, -37.9052)
  line L226 (69.0555, -46.7975) -> (67.8055, -48.9625) construction
  line L227 (69.0555, -46.7975) -> (67.8055, -48.9625) construction
  line L228 (72.0555, -41.6013) -> (69.0555, -46.7975)
  line L229 (74.6535, -43.1013) -> (71.6536, -48.2974)
  line L230 (69.0555, -46.7975) -> (69.4896, -49.2595)
  line L231 (71.6536, -48.2974) -> (70.6536, -50.0295) construction
  line L232 (71.6536, -48.2974) -> (72.0008, -50.2671)
  line L233 (69.4896, -49.2595) -> (65.9896, -55.3217)
  line L234 (72.0008, -50.2671) -> (69.5008, -54.5972)
  line L235 (69.5008, -54.5972) -> (77.0008, -67.5876)
  line L236 (65.9896, -55.3217) -> (75.9896, -72.6422)
  line L237 (70.967, -58.1954) -> (60.967, -75.5159) construction
  line L238 (81.9249, -66.7193) -> (83.4249, -64.1213)
  line L239 (84.8529, -71.0793) -> (87.7429, -66.0737)
  line L240 (87.7429, -66.0737) -> (85.4929, -69.9708) construction
  line L241 (87.7429, -66.0737) -> (85.4929, -62.1766)
  line L242 (83.4249, -64.1213) -> (82.1749, -61.9562)
  line L243 (77.0008, -67.5876) -> (81.9249, -66.7193)
  line L244 (75.9896, -72.6422) -> (84.8529, -71.0793)
  line L245 (96.5929, 42.9507) -> (91.0429, 52.5636)
  line L246 (94.743, 40.1874) -> (88.4589, 51.0717)
  line L247 (82.1749, 61.956) -> (88.4589, 51.0717)
  line L248 (85.4929, 62.1765) -> (91.0429, 52.5636)
  line L249 (87.7429, 66.0736) -> (85.4929, 62.1765)
  line L250 (83.4249, 64.1211) -> (82.1749, 61.956)
  line L251 (75.9896, 72.642) -> (84.8529, 71.0793)
  line L252 (87.7429, 66.0736) -> (85.4929, 69.9707) construction
  line L253 (84.8529, 71.0793) -> (87.7429, 66.0736)
  line L254 (81.9249, 66.7192) -> (83.4249, 64.1211)
  line L255 (77.0008, 67.5874) -> (81.9249, 66.7192)
  line L256 (65.9896, 55.3215) -> (75.9896, 72.642)
  line L257 (69.5008, 54.597) -> (77.0008, 67.5874)
  line L258 (72.0008, 50.2669) -> (69.5008, 54.597)
  line L259 (69.4896, 49.2593) -> (65.9896, 55.3215)
  line L260 (71.6536, 48.2973) -> (72.0008, 50.2669)
  line L261 (69.0555, 46.7973) -> (69.4896, 49.2593)
  line L262 (69.0555, 46.7973) -> (67.8054, 48.9624) construction
  line L263 (69.0555, 46.7973) -> (67.8055, 48.9624) construction
  line L264 (72.0555, 41.6012) -> (69.0555, 46.7973)
  line L265 (71.6536, 48.2973) -> (70.6536, 50.0293) construction
  line L266 (74.6535, 43.1012) -> (71.6536, 48.2973)
  line L267 (75.0555, 36.4051) -> (76.3055, 34.24) construction
  line L268 (75.0555, 36.4051) -> (76.3055, 34.24) construction
  line L269 (72.0555, 41.6012) -> (75.0555, 36.4051)
  line L270 (74.6535, 43.1012) -> (77.6535, 37.9051)
  line L271 (75.0555, 36.4051) -> (77.4047, 35.55)
  line L272 (77.6535, 37.9051) -> (78.6535, 36.173) construction
  line L273 (77.6535, 37.9051) -> (79.5329, 37.221)
  line L274 (77.4047, 35.55) -> (80.9047, 29.4879)
  line L275 (79.5329, 37.221) -> (82.0329, 32.8909)
  line L276 (82.0329, 32.8909) -> (97.0329, 32.8909)
  line L277 (80.9047, 29.4879) -> (100.9047, 29.4879)
  line L278 (85.8821, 32.3615) -> (95.8821, 15.041) construction
  line L279 (98.743, 37.5894) -> (97.243, 40.1874)
  line L280 (103.9829, 37.9451) -> (101.0929, 42.9507)
  line L281 (101.0929, 42.9507) -> (103.3429, 39.0536) construction
  line L282 (101.0929, 42.9507) -> (96.5929, 42.9507)
  line L283 (97.243, 40.1874) -> (94.743, 40.1874)
  line L284 (97.0329, 32.8909) -> (98.743, 37.5894)
  line L285 (100.9047, 29.4879) -> (103.9829, 37.9451)
  line L286 (11.0999, 105.1272) -> (-0.0001, 105.1272)
  line L287 (12.5681, 102.1435) -> (0, 102.1435)
  line L288 (-12.5681, 102.1435) -> (0, 102.1435)
  line L289 (-11.1001, 105.1272) -> (-0.0001, 105.1272)
  line L290 (-13.3501, 109.0244) -> (-11.1001, 105.1272)
  line L291 (-13.8181, 104.3086) -> (-12.5681, 102.1435)
  line L292 (-24.9151, 102.1299) -> (-19.1301, 109.0244)
  line L293 (-13.3501, 109.0244) -> (-17.8501, 109.0244) construction
  line L294 (-19.1301, 109.0244) -> (-13.3501, 109.0244)
  line L295 (-16.8181, 104.3086) -> (-13.8181, 104.3086)
  line L296 (-20.0321, 100.4784) -> (-16.8181, 104.3086)
  line L297 (-14.9151, 84.8094) -> (-24.9151, 102.1299)
  line L298 (-12.5321, 87.488) -> (-20.0321, 100.4784)
  line L299 (-7.5321, 87.488) -> (-12.5321, 87.488)
  line L300 (-7.9151, 84.8094) -> (-14.9151, 84.8094)
  line L301 (-6, 86.2024) -> (-7.5321, 87.488)
  line L302 (-6, 83.2024) -> (-7.9151, 84.8094)
  line L303 (-6, 83.2024) -> (-8.5001, 83.2024) construction
  line L304 (-6, 83.2024) -> (-8.5, 83.2024) construction
  line L305 (0, 83.2024) -> (-6, 83.2024)
  line L306 (-6, 86.2024) -> (-8, 86.2024) construction
  line L307 (0, 86.2024) -> (-6, 86.2024)
  line L308 (5.9999, 83.2025) -> (8.4999, 83.2025) construction
  line L309 (5.9999, 83.2025) -> (8.4999, 83.2025) construction
  line L310 (0, 83.2024) -> (5.9999, 83.2025)
  line L311 (0, 86.2024) -> (5.9999, 86.2024)
  line L312 (5.9999, 83.2025) -> (7.915, 84.8094)
  line L313 (5.9999, 86.2024) -> (7.9999, 86.2024) construction
  line L314 (5.9999, 86.2024) -> (7.532, 87.488)
  line L315 (7.915, 84.8094) -> (14.915, 84.8094)
  line L316 (7.532, 87.488) -> (12.532, 87.488)
  line L317 (12.532, 87.488) -> (20.032, 100.4784)
  line L318 (14.915, 84.8094) -> (24.915, 102.13)